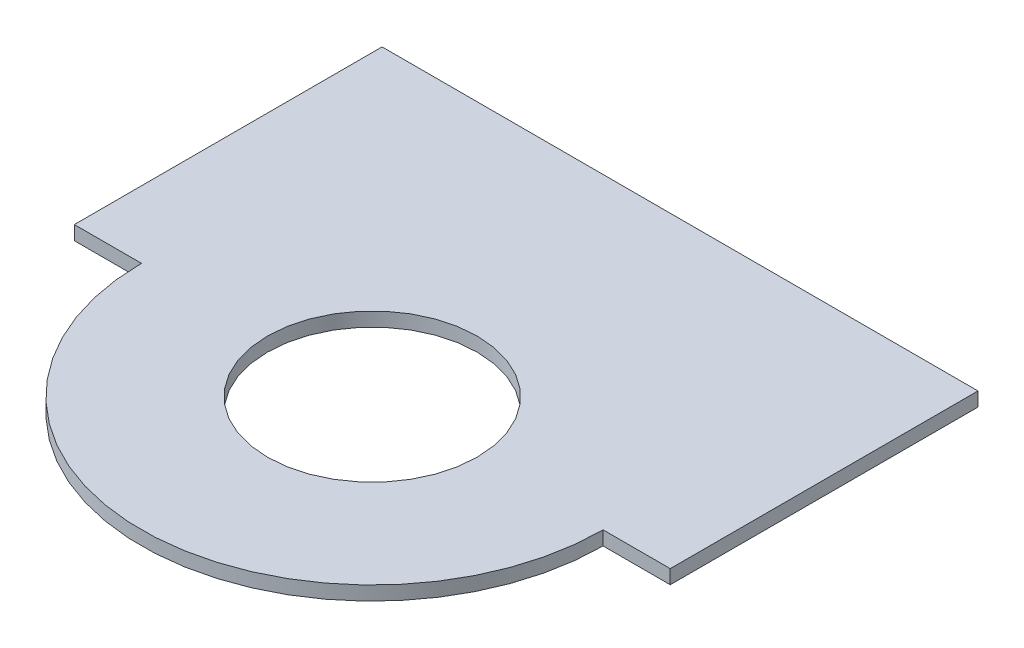
# Autodesk Inventor part: frontPlate_half
Saved by Autodesk Inventor 2014 SP1 (Build 180222100, 222)
## iProperties
Created: 2015-02-25
Part Number: frontPlate_half
Material: Generic
Document SubType Name: Modeling
Designer: Simen
Density: 1 g/cm^3
Appearance: Default
Author: Simen
Autodesk Inventor part; units mm, degrees
ref_plane "YZ Plane" through (0, 0, 0) normal (1, 0, 0) x (0, 1, 0)
ref_plane "XZ Plane" through (0, 0, 0) normal (0, 1, 0) x (-1, 0, 0)
ref_plane "XY Plane" through (0, 0, 0) normal (0, 0, 1) x (1, 0, 0)
sketch "Sketch1" plane through (0, 0, 0) normal (0, 1, 0) x (-1, 0, 0)
  line L0 (341.2381, 167.58) -> (341.2381, -52.42)
  line L1 (341.2381, -52.42) -> (-84.7619, -52.42)
  line L2 (-84.7619, -52.42) -> (-84.7619, 167.58)
  arc A0 (293.2381, 167.58) -> (-36.7619, 167.58) centre (128.2381, 167.58) ccw
  line L3 (-84.7619, 167.58) -> (-36.7619, 167.58)
  line L4 (293.2381, 167.58) -> (341.2381, 167.58)
  circle A1 centre (128.2381, 167.58) radius 75
  point P0 (0, 0)
  dimension "d0" = 426
  dimension "d1" = 220
  dimension "d2" = 330
  dimension "d3" = 150
  constraints: 10 end point, 3 parallel, 2 centre point, 2 horizontal, 2 perpendicular, 2 point on circle, 1 coincident
  measures "d0" distance of L0.end L1.end
  measures "d1" distance of L0.start L0.end
  measures "d2" diameter of A0
  measures "d3" diameter of A1
extrude "Extrusion1" add sketch "Sketch1" along normal blind 10
body "Solid1"
